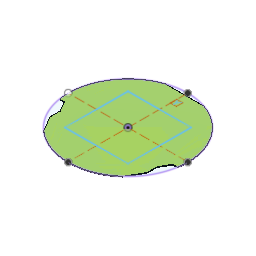
bed_shape (Autodesk Fusion 360 design; units mm, degrees)
Autodesk Fusion 360 part; units mm, degrees
sketch "Sketch1" plane through (0, 0, 0) normal (0, 0, 1) x (1, 0, 0)
  circle A0 centre (0, 0) radius 95
  line L0 (0, 0) -> (120, 0) construction
  line L1 (0, 0) -> (103.923, -60) construction
  line L2 (0, 0) -> (120, 0) construction
  line L3 (30.4138, 90) -> (-30.4138, 90)
  line L4 (62.7354, -71.3391) -> (93.1492, -18.6609)
  line L5 (0, -100) -> (0, 100) construction
  line L6 (76.923, -15) -> (103.923, -15)
  line L7 (103.923, -15) -> (103.923, -60) construction
  line L8 (103.923, -60) -> (76.923, -60) construction
  line L9 (76.923, -60) -> (76.923, -15)
  circle A1 centre (0, 0) radius 120 construction
  line L10 (76.923, -30.7654) -> (86.0252, -15)
  line L11 (-76.923, -30.7654) -> (-86.0252, -15)
  line L12 (-62.7354, -71.3391) -> (-93.1492, -18.6609)
  line L13 (-76.923, -60) -> (-76.923, -15)
  line L14 (-76.923, -15) -> (-103.923, -15)
  line L15 (-24, -91.9184) -> (-24, -75)
  line L16 (-24, -75) -> (24, -75)
  line L17 (24, -75) -> (24, -91.9184)
  line L18 (-87.9147, 36) -> (-77, 36)
  line L19 (-77, 36) -> (-58, 69)
  line L20 (-58, 69) -> (-58, 75.2396)
  line L21 (56, 76.7398) -> (56, 59)
  line L22 (56, 59) -> (78, 38)
  line L23 (78, 38) -> (87.0689, 38)
  dimension "d1" = 190
  dimension "d5" = 30
  dimension "d14" = 90
  dimension "d15" = 90
  dimension "d18" = 240
  dimension "d19" = 27
  dimension "d20" = 45
  dimension "d22" = 8
  dimension "d24" = 12
  dimension "d25" = 78.923
  dimension "d26" = 83.5117
  dimension "d30" = 86.0252
  dimension "d31" = 30.7654
  dimension "d32" = 48
  dimension "d33" = 75
  dimension "d34" = 58
  dimension "d35" = 36
  dimension "d36" = 77
  dimension "d37" = 69
  dimension "d38" = 38
  dimension "d39" = 78
  dimension "d40" = 56
  dimension "d41" = 59
  constraint coincident A0.centre L0.start
  constraint horizontal L0
  constraint horizontal L2
  constraint horizontal L3
  constraint coincident A0 L4.start
  constraint coincident A0 L4.end
  constraint perpendicular L1 L4
  constraint vertical L5
  constraint coincident A0 L3.end
  constraint coincident A0 L3.start
  constraint horizontal L6
  constraint vertical L7
  constraint horizontal L8
  constraint vertical L9
  constraint concentric A0 A1
  constraint coincident L1.end A1
  constraint parallel L4 L10
  constraint coincident L6 L10.end
  constraint coincident L9 L10.start
  constraint symmetric L4.start L5 L12.start
  constraint symmetric L4.end L5 L12.end
  constraint symmetric L5 L6.start L13.end
  constraint symmetric L5 L6.end L14.end
  constraint symmetric L5 L8.end L13.start
  constraint symmetric L5 L10.end L11.end
  constraint symmetric L5 L10.start L11.start
  constraint coincident A0 L15.start
  constraint vertical L15
  constraint perpendicular L15 L16
  constraint coincident A0 L17.end
  constraint perpendicular L16 L17
  constraint symmetric L5 L15 L17
  constraint coincident A0 L18.start
  constraint horizontal L18
  constraint coincident A0 L20.end
  constraint perpendicular L18 L20
  constraint coincident A0 L21.start
  constraint vertical L21
  constraint coincident A0 L23.end
  constraint horizontal L23
  measures "d1" diameter of A0
  measures "d5" angle of L1 L2
  measures "d14" distance of A0.centre L3
  measures "d15" distance of A0.centre L4
  measures "d18" diameter of A1
  measures "d19" distance of L1.end L8.end
  measures "d20" distance of L1.end L6.end
  measures "d22" distance of L4 L10
  measures "d30" horizontal distance of A0.centre L10.end
  measures "d31" vertical distance of A0.centre L10.start
  measures "d32" distance of L15.end L16.end
  measures "d33" distance of A0.centre L16
  measures "d34" distance of L5 L20
  measures "d35" distance of A0.centre L18
  measures "d36" distance of L5 L18.end
  measures "d37" vertical distance of A0.centre L19.end
  measures "d38" distance of L0 L23
  measures "d39" distance of L5 L22.end
  measures "d40" distance of L5 L21
  measures "d41" distance of L0 L21.end
extrude "Extrude1" add sketch "Sketch1" along normal blind 1 contours A0 L3 L4 L6 L9 L12 L13 L14 L15 L16 L17 L18 L19 L20 L21 L22 L23 | A0 L21 L22 L23 | L6 L9 L10 | A0 L18 L19 L20 | A0 L15 L16 L17 | L11 L13 L14
sketch "Sketch2" plane through (0, 0, 1) normal (0, 0, 1) x (-1, 0, 0)
  line L0 (-30.4138, -90) -> (30.4138, -90)
  arc A0 (30.4138, -90) -> (93.8083, 15) centre (0, 0) ccw
  line L1 (93.8083, 15) -> (86.0252, 15)
  line L2 (86.0252, 15) -> (76.923, 30.7654)
  line L3 (76.923, 30.7654) -> (76.923, 46.7654)
  line L4 (76.923, 46.7654) -> (62.7354, 71.3391)
  arc A1 (62.7354, 71.3391) -> (-62.7354, 71.3391) centre (0, 0) ccw
  line L5 (-62.7354, 71.3391) -> (-76.923, 46.7654)
  line L6 (-76.923, 46.7654) -> (-76.923, 30.7654)
  line L7 (-76.923, 30.7654) -> (-86.0252, 15)
  line L8 (-86.0252, 15) -> (-93.8083, 15)
  arc A2 (-93.8083, 15) -> (-30.4138, -90) centre (0, 0) ccw
  circle A3 centre (0, 0) radius 95
  line L9 (50, -50) -> (-50, -50)
  line L10 (0, -95) -> (0, 95) construction
  line L11 (-95, 0) -> (95, 0) construction
  line L12 (50, 50) -> (-50, 50)
  line L13 (-50, -50) -> (-50, 50)
  line L14 (50, -50) -> (50, 50)
  line L15 (0.0222, -67.584) -> (-9.3085, -67.5632) construction
  line L16 (-9.3085, -67.5632) -> (-9.3307, -77.4981) construction
  line L17 (-9.3307, -77.4981) -> (0, -77.5189) construction
  line L18 (0, -77.5189) -> (0.0222, -67.584) construction
  dimension "d42" = 100
  dimension "d43" = 100
  constraint horizontal L9
  constraint coincident A3 L10.start
  constraint coincident A3 L10.end
  constraint coincident A2 L11.start
  constraint coincident A0.centre L10
  constraint coincident A0.centre L11
  constraint symmetric L9.start L11 L12.start
  constraint symmetric L9.end L11 L12.end
  constraint coincident L10
  measures "d42" distance of L9.start L9.end
  measures "d43" distance of L9.start L12.start
